LGR Height Extension (Autodesk Fusion 360 design; units mm, degrees)
Autodesk Fusion 360 part; units mm, degrees
note: some values were not read from the file. Set by a fixed rule: which sketch regions a step uses.
sketch "Sketch1" plane through (0, 0, 0) normal (0, 0, 1) x (1, 0, 0)
  line L0 (-28.575, 22.5) -> (28.575, 22.5)
  line L1 (28.575, 22.5) -> (28.575, -22.5)
  line L2 (28.575, -22.5) -> (-28.575, -22.5)
  line L3 (-28.575, -22.5) -> (-28.575, 22.5)
  dimension "d1" = 45
  dimension "d2" = 57.15
  dimension "d7" = 28.575
  dimension "d8" = 22.5
  constraint horizontal L0
  constraint vertical L1
  constraint horizontal L2
  constraint vertical L3
  measures "d1" distance of L0 L2
  measures "d2" distance of L1 L3
  measures "d7" distance of origin L1
  measures "d8" distance of origin L0
extrude "Extrude1" add sketch "Sketch1" along normal blind 1 makes body 1
sketch "Sketch3" plane through (0, 0, 1) normal (0, 0, 1) x (-1, 0, 0)
  line L0 (28.575, 22.5) -> (-28.575, 22.5)
  line L1 (-28.575, 22.5) -> (-28.575, -22.5)
  line L2 (-28.575, -22.5) -> (28.575, -22.5)
  line L3 (28.575, -22.5) -> (28.575, 22.5)
  line L4 (28.575, -22.5) -> (-28.575, -22.5)
  line L5 (-28.575, -22.5) -> (-28.575, -23.5)
  line L6 (-28.575, -23.5) -> (28.575, -23.5)
  line L7 (28.575, -23.5) -> (28.575, -22.5)
  dimension "d9" = 1
  dimension "d10" = 57.15
  constraint horizontal L4
  constraint vertical L5
  constraint horizontal L6
  constraint vertical L7
  constraint coincident L2.end L3.start
  measures "d9" distance of L4 L6
  measures "d10" distance of L5 L7
extrude "Extrude2" add sketch "Sketch3" along normal blind 45 separate body contours L2 L4 L5 L6 L7 makes body 2
extrude "Extrude3" add 1 faces at (-9.525, 23.1667, 1) along direction (0, 0, -1) blind 1 on bodies 2 bodies 1 2
extrude "Extrude4" add 1 faces at (9.525, 23.5, 30.6667) along direction (0, 1, 0) blind 5 on bodies 1 bodies 1
extrude "Extrude5" add 1 faces at (-9.525, 11.5, 0) along direction (0, 0, -1) blind 5 on bodies 1 bodies 1
sketch "Sketch5" plane through (0, 28.5, 0) normal (0, 1, 0) x (-1, 0, 0)
  line L0 (28.575, -5) -> (28.575, 46)
  line L1 (28.575, 46) -> (-28.575, 46)
  line L2 (-28.575, 46) -> (-28.575, -5)
  line L3 (-28.575, -5) -> (28.575, -5)
  point P0 (-20, 30.5)
  point P1 (20, 30.5)
  point P2 (-20, 18.5)
  point P3 (20, 18.5)
  dimension "d28" = 40
  dimension "d29" = 12
  dimension "d31" = 8.575
  dimension "d38" = 23.5
  constraint horizontal P0 P1
  constraint vertical P1 P3
  constraint horizontal P2 P3
  constraint vertical P0 P2
  measures "d28" distance of P0 P1
  measures "d29" distance of P1 P3
  measures "d31" distance of L2 P0
  measures "d38" distance of L3 P2
hole "Hole2" at (20, 28.5, 30.5) at (-20, 28.5, 30.5) at (-20, 28.5, 18.5) at (20, 28.5, 18.5) direction (0, -1, 0) diameter 5.5 depth 6 tip angle 180 counterbore diameter 10 counterbore depth 5 bodies 1
extrude "Extrude6" cut 1 faces at (-28.575, 9.5, -3) along direction (-1, 0, 0) blind 0 and the other way blind 2 on bodies 1 bodies 1
extrude "Extrude7" cut 1 faces at (28.575, 9.5, -3) along direction (1, 0, 0) blind 0 and the other way blind 2 on bodies 1 bodies 1
extrude "Extrude8" cut 1 faces at (-8.8583, 24.5, 46) along direction (0, 0, 1) blind 0 and the other way blind 7.5 on bodies 1 bodies 1
sketch "Sketch6" plane through (0, 28.5, 0) normal (0, 1, 0) x (-1, 0, 0)
  line L0 (26.575, 38.5) -> (-26.575, 38.5)
  line L1 (-26.575, 38.5) -> (-26.575, -5)
  line L2 (-26.575, -5) -> (26.575, -5)
  line L3 (26.575, -5) -> (26.575, 38.5)
  circle A0 centre (20, 18.5) radius 5
  circle A1 centre (-20, 30.5) radius 5
  circle A2 centre (20, 30.5) radius 5
  circle A3 centre (-20, 18.5) radius 5
  circle A4 centre (0, 24.5) radius 12.5
  dimension "d51" = 25
  dimension "d52" = 20
  dimension "d53" = 6
  measures "d51" diameter of A4
  measures "d52" horizontal distance of A3.centre A4.centre
  measures "d53" vertical distance of A2.centre A4.centre
extrude "Extrude9" cut sketch "Sketch6" along normal blind 0 and the other way blind 6 contours A4 bodies 1
sketch "Sketch9" plane through (0, 0, 1) normal (0, 0, 1) x (-1, 0, 0)
  line L0 (-26.575, 22.5) -> (-26.575, -22.5)
  line L1 (-26.575, -22.5) -> (26.575, -22.5)
  line L2 (26.575, -22.5) -> (26.575, 22.5)
  line L3 (26.575, 22.5) -> (-26.575, 22.5)
  line L4 (16.3972, -20) -> (-16.3972, -20)
  line L5 (24.075, -13.7886) -> (24.075, 13.7886)
  line L6 (16.3972, 20) -> (-16.3972, 20)
  line L7 (-24.075, 13.7886) -> (-24.075, -13.7886)
  line L8 (-1.2665, -3.0362) -> (-17.6637, -16.4521)
  line L9 (1.2665, -3.0362) -> (17.6637, -16.4521)
  line L10 (20.8111, -15.3386) -> (3.9009, -1.55)
  line L11 (3.9009, 1.55) -> (20.8111, 15.3386)
  line L12 (17.6637, 16.4521) -> (1.2665, 3.0362)
  line L13 (-1.2665, 3.0362) -> (-17.6637, 16.4521)
  line L14 (-20.8111, 15.3386) -> (-3.9009, 1.55)
  line L15 (-3.9009, -1.55) -> (-20.8111, -15.3386)
  arc A0 (20.8111, -15.3386) -> (24.075, -13.7886) centre (22.075, -13.7886) ccw
  arc A1 (3.9009, 1.55) -> (3.9009, -1.55) centre (5.1648, 0) ccw
  arc A2 (24.075, 13.7886) -> (20.8111, 15.3386) centre (22.075, 13.7886) ccw
  arc A3 (17.6637, 16.4521) -> (16.3972, 20) centre (16.3972, 18) ccw
  arc A4 (-16.3972, 20) -> (-17.6637, 16.4521) centre (-16.3972, 18) ccw
  arc A5 (-1.2665, 3.0362) -> (1.2665, 3.0362) centre (0, 4.5841) ccw
  arc A6 (-3.9009, -1.55) -> (-3.9009, 1.55) centre (-5.1648, 0) ccw
  arc A7 (-20.8111, 15.3386) -> (-24.075, 13.7886) centre (-22.075, 13.7886) ccw
  arc A8 (-24.075, -13.7886) -> (-20.8111, -15.3386) centre (-22.075, -13.7886) ccw
  arc A9 (-17.6637, -16.4521) -> (-16.3972, -20) centre (-16.3972, -18) ccw
  arc A10 (16.3972, -20) -> (17.6637, -16.4521) centre (16.3972, -18) ccw
  arc A11 (1.2665, -3.0362) -> (-1.2665, -3.0362) centre (0, -4.5841) ccw
  point P0 (22, -20)
  point P1 (-22, -20)
  point P2 (24.075, -18)
  point P3 (24.075, 18)
  point P4 (22, 20)
  point P5 (-22, 20)
  point P6 (-24.075, 18)
  point P7 (-24.075, -18)
  point P8 (0, -2)
  point P9 (-2, 0)
  point P10 (0, 2)
  point P11 (2, 0)
  dimension "d93" = 44
  dimension "d94" = 44
  dimension "d95" = 36
  dimension "d96" = 36
  dimension "d97" = 22
  dimension "d98" = 22
  dimension "d99" = 18
  dimension "d100" = 18
  dimension "d101" = 2.5
  dimension "d102" = 2.5
  dimension "d103" = 2.5
  dimension "d104" = 2.5
  dimension "d105" = 2
  dimension "d112" = 2
  constraint horizontal L4
  constraint parallel L2 L5
  constraint horizontal L6
  constraint parallel L0 L7
  constraint coincident P2 L10
  constraint coincident P2 L5
  constraint tangent L10 A0
  constraint tangent L5 A0
  constraint tangent L10 A1
  constraint tangent L11 A1
  constraint equal A0 A1
  constraint coincident P3 L11
  constraint coincident P3 L5
  constraint tangent L11 A2
  constraint tangent L5 A2
  constraint equal A0 A2
  constraint coincident P4 L12
  constraint coincident P4 L6
  constraint tangent L12 A3
  constraint tangent L6 A3
  constraint equal A0 A3
  constraint coincident P5 L6
  constraint coincident P5 L13
  constraint tangent L6 A4
  constraint tangent L13 A4
  constraint equal A0 A4
  constraint tangent L13 A5
  constraint tangent L12 A5
  constraint equal A0 A5
  constraint tangent L14 A6
  constraint tangent L15 A6
  constraint equal A0 A6
  constraint coincident P6 L14
  constraint coincident P6 L7
  constraint tangent L14 A7
  constraint tangent L7 A7
  constraint equal A0 A7
  constraint coincident P7 L7
  constraint coincident P7 L15
  constraint tangent L7 A8
  constraint tangent L15 A8
  constraint equal A0 A8
  constraint coincident P1 L8
  constraint coincident P1 L4
  constraint tangent L8 A9
  constraint tangent L4 A9
  constraint equal A0 A9
  constraint coincident P0 L9
  constraint coincident P0 L4
  constraint tangent L9 A10
  constraint tangent L4 A10
  constraint equal A0 A10
  constraint tangent L9 A11
  constraint tangent L8 A11
  measures "d93" distance of P0 P1
  measures "d94" distance of P4 P5
  measures "d95" distance of P6 P7
  measures "d96" distance of P2 P3
  measures "d97" horizontal distance of origin P1
  measures "d98" horizontal distance of origin P4
  measures "d99" vertical distance of origin P6
  measures "d100" vertical distance of origin P2
  measures "d101" distance of L3 L6
  measures "d102" distance of L0 L7
  measures "d103" distance of L2 L5
  measures "d104" distance of L1 L4
  measures "d105" radius of A0
  measures "d112" radius of A11
extrude "Extrude11" cut sketch "Sketch9" along normal blind 0 and the other way blind 6 contours L4 L8 L9 A9 A10 A11 | L5 L10 L11 A0 A1 A2 | L6 L12 L13 A3 A4 A5 | L7 L14 L15 A6 A7 A8 bodies 1
sketch "Sketch10" plane through (0, 22.5, 0) normal (0, -1, 0) x (1, 0, 0)
  circle A0 centre (0, 24.5) radius 12.5
  line L0 (26.575, 38.5) -> (-26.575, 38.5)
  line L1 (-26.575, 38.5) -> (-26.575, 1)
  line L2 (-26.575, 1) -> (26.575, 1)
  line L3 (26.575, 1) -> (26.575, 38.5)
  circle A1 centre (20, 18.5) radius 2.75
  circle A2 centre (-20, 30.5) radius 2.75
  circle A3 centre (20, 30.5) radius 2.75
  circle A4 centre (-20, 18.5) radius 2.75
  line L4 (-21.575, 9.5) -> (21.575, 9.5)
  line L5 (24.075, 7) -> (24.075, 6)
  line L6 (21.575, 3.5) -> (-21.575, 3.5)
  line L7 (-24.075, 6) -> (-24.075, 7)
  arc A5 (-21.575, 9.5) -> (-24.075, 7) centre (-21.575, 7) ccw
  arc A6 (-24.075, 6) -> (-21.575, 3.5) centre (-21.575, 6) ccw
  arc A7 (21.575, 3.5) -> (24.075, 6) centre (21.575, 6) ccw
  arc A8 (24.075, 7) -> (21.575, 9.5) centre (21.575, 7) ccw
  dimension "d113" = 2.5
  dimension "d114" = 2.5
  dimension "d115" = 2.5
  dimension "d116" = 15
  dimension "d117" = 2.5
  constraint horizontal L4
  constraint vertical L5
  constraint horizontal L6
  constraint vertical L7
  constraint tangent L4 A5
  constraint tangent L7 A5
  constraint tangent L7 A6
  constraint tangent L6 A6
  constraint equal A5 A6
  constraint tangent L6 A7
  constraint tangent L5 A7
  constraint equal A5 A7
  constraint tangent L5 A8
  constraint tangent L4 A8
  constraint equal A5 A8
  measures "d113" distance of L2 L6
  measures "d114" distance of L1 L7
  measures "d115" distance of L3 L5
  measures "d116" distance of A0.centre L4
  measures "d117" radius of A5
extrude "Extrude13" cut sketch "Sketch10" against normal blind 6 contours L4 L5 L6 L7 A5 A6 A7 A8 bodies 1
extrude "Extrude14" add 1 faces at (5.4657, 25.6667, -5) along direction (0, 0, -1) blind 5 on bodies 1 bodies 1
sketch "Sketch13" plane through (26.575, 0, 0) normal (1, 0, 0) x (0, 1, 0)
  line L0 (28.5, 38.5) -> (22.5, 38.5)
  line L1 (22.5, 38.5) -> (22.5, 1)
  line L2 (22.5, 1) -> (-22.5, 1)
  line L3 (-22.5, 1) -> (-22.5, -10)
  line L4 (-22.5, -10) -> (28.5, -10)
  line L5 (28.5, -10) -> (28.5, 38.5)
  line L6 (-13, -1.5) -> (13, -1.5)
  line L7 (15, -3.5) -> (15, -5.5)
  line L8 (13, -7.5) -> (-13, -7.5)
  line L9 (-15, -5.5) -> (-15, -3.5)
  arc A0 (-13, -1.5) -> (-15, -3.5) centre (-13, -3.5) ccw
  arc A1 (-15, -5.5) -> (-13, -7.5) centre (-13, -5.5) ccw
  arc A2 (13, -7.5) -> (15, -5.5) centre (13, -5.5) ccw
  arc A3 (15, -3.5) -> (13, -1.5) centre (13, -3.5) ccw
  dimension "d124" = 2.5
  dimension "d125" = 2.5
  dimension "d126" = 7.5
  dimension "d127" = 13.5
  dimension "d128" = 2
  constraint horizontal L6
  constraint vertical L7
  constraint horizontal L8
  constraint vertical L9
  constraint tangent L6 A0
  constraint tangent L9 A0
  constraint tangent L9 A1
  constraint tangent L8 A1
  constraint equal A0 A1
  constraint tangent L8 A2
  constraint tangent L7 A2
  constraint equal A0 A2
  constraint tangent L7 A3
  constraint tangent L6 A3
  constraint equal A0 A3
  measures "d124" distance of L2 L6
  measures "d125" distance of L4 L8
  measures "d126" distance of L3 L9
  measures "d127" distance of L5 L7
  measures "d128" radius of A0
extrude "Extrude15" cut sketch "Sketch13" against normal blind 4 contours L6 L7 L8 L9 A0 A1 A2 A3 bodies 1
sketch "Sketch14" plane through (0, -22.5, 0) normal (0, -1, 0) x (1, 0, 0)
  line L0 (26.575, -10) -> (26.575, 1)
  line L1 (26.575, 1) -> (-26.575, 1)
  line L2 (-26.575, 1) -> (-26.575, -10)
  line L3 (-26.575, -10) -> (26.575, -10)
  line L4 (-15.5, -1.5) -> (15.5, -1.5)
  line L5 (17.5, -3.5) -> (17.5, -5.5)
  line L6 (15.5, -7.5) -> (-15.5, -7.5)
  line L7 (-17.5, -5.5) -> (-17.5, -3.5)
  arc A0 (-15.5, -1.5) -> (-17.5, -3.5) centre (-15.5, -3.5) ccw
  arc A1 (-17.5, -5.5) -> (-15.5, -7.5) centre (-15.5, -5.5) ccw
  arc A2 (15.5, -7.5) -> (17.5, -5.5) centre (15.5, -5.5) ccw
  arc A3 (17.5, -3.5) -> (15.5, -1.5) centre (15.5, -3.5) ccw
  dimension "d131" = 2.5
  dimension "d132" = 2.5
  dimension "d133" = 9.075
  dimension "d134" = 9.075
  dimension "d135" = 2
  constraint horizontal L4
  constraint vertical L5
  constraint horizontal L6
  constraint vertical L7
  constraint tangent L4 A0
  constraint tangent L7 A0
  constraint tangent L7 A1
  constraint tangent L6 A1
  constraint equal A0 A1
  constraint tangent L6 A2
  constraint tangent L5 A2
  constraint equal A0 A2
  constraint tangent L4 A3
  constraint tangent L5 A3
  constraint equal A0 A3
  measures "d131" distance of L1 L4
  measures "d132" distance of L3 L6
  measures "d133" distance of L2 L7
  measures "d134" distance of L0 L5
  measures "d135" radius of A0
extrude "Extrude16" cut sketch "Sketch14" against normal blind 4 contours L4 L5 L6 L7 A0 A1 A2 A3 bodies 1
sketch "Sketch15" plane through (-26.575, 0, 0) normal (-1, 0, 0) x (0, -1, 0)
  line L0 (-22.5, 38.5) -> (-28.5, 38.5)
  line L1 (-28.5, 38.5) -> (-28.5, -10)
  line L2 (-28.5, -10) -> (22.5, -10)
  line L3 (22.5, -10) -> (22.5, 1)
  line L4 (22.5, 1) -> (-22.5, 1)
  line L5 (-22.5, 1) -> (-22.5, 38.5)
  line L6 (-13, -1.5) -> (13, -1.5)
  line L7 (15, -3.5) -> (15, -5.5)
  line L8 (13, -7.5) -> (-13, -7.5)
  line L9 (-15, -5.5) -> (-15, -3.5)
  arc A0 (15, -3.5) -> (13, -1.5) centre (13, -3.5) ccw
  arc A1 (13, -7.5) -> (15, -5.5) centre (13, -5.5) ccw
  arc A2 (-15, -5.5) -> (-13, -7.5) centre (-13, -5.5) ccw
  arc A3 (-13, -1.5) -> (-15, -3.5) centre (-13, -3.5) ccw
  dimension "d138" = 2.5
  dimension "d139" = 2.5
  dimension "d140" = 7.5
  dimension "d141" = 13.5
  dimension "d142" = 2
  constraint horizontal L6
  constraint vertical L7
  constraint horizontal L8
  constraint vertical L9
  constraint tangent L7 A0
  constraint tangent L6 A0
  constraint tangent L7 A1
  constraint tangent L8 A1
  constraint equal A0 A1
  constraint tangent L8 A2
  constraint tangent L9 A2
  constraint equal A0 A2
  constraint tangent L9 A3
  constraint tangent L6 A3
  constraint equal A0 A3
  measures "d138" distance of L4 L6
  measures "d139" distance of L2 L8
  measures "d140" distance of L3 L7
  measures "d141" distance of L1 L9
  measures "d142" radius of A0
extrude "Extrude17" cut sketch "Sketch15" against normal blind 4 contours L6 L7 L8 L9 A0 A1 A2 A3 bodies 1
sketch "Sketch16" plane through (0, 28.5, 0) normal (0, 1, 0) x (-1, 0, 0)
  line L0 (-24.075, 6) -> (-24.075, 7)
  arc A0 (-21.575, 9.5) -> (-24.075, 7) centre (-21.575, 7) ccw
  line L1 (-21.575, 9.5) -> (21.575, 9.5)
  arc A1 (24.075, 7) -> (21.575, 9.5) centre (21.575, 7) ccw
  line L2 (24.075, 7) -> (24.075, 6)
  arc A2 (21.575, 3.5) -> (24.075, 6) centre (21.575, 6) ccw
  line L3 (21.575, 3.5) -> (-21.575, 3.5)
  arc A3 (-24.075, 6) -> (-21.575, 3.5) centre (-21.575, 6) ccw
  circle A4 centre (0, 24.5) radius 12.5
  line L4 (26.575, 38.5) -> (-26.575, 38.5)
  line L5 (-26.575, 38.5) -> (-26.575, -10)
  line L6 (-26.575, -10) -> (26.575, -10)
  line L7 (26.575, -10) -> (26.575, 38.5)
  circle A5 centre (20, 18.5) radius 5
  circle A6 centre (-20, 30.5) radius 5
  circle A7 centre (20, 30.5) radius 5
  circle A8 centre (-20, 18.5) radius 5
  line L8 (-15.5, -1.5) -> (15.5, -1.5)
  line L9 (17.5, -3.5) -> (17.5, -5.5)
  line L10 (15.5, -7.5) -> (-15.5, -7.5)
  line L11 (-17.5, -5.5) -> (-17.5, -3.5)
  arc A9 (-15.5, -1.5) -> (-17.5, -3.5) centre (-15.5, -3.5) ccw
  arc A10 (-17.5, -5.5) -> (-15.5, -7.5) centre (-15.5, -5.5) ccw
  arc A11 (15.5, -7.5) -> (17.5, -5.5) centre (15.5, -5.5) ccw
  arc A12 (17.5, -3.5) -> (15.5, -1.5) centre (15.5, -3.5) ccw
  dimension "d145" = 5
  dimension "d146" = 2.5
  dimension "d147" = 9.075
  dimension "d148" = 9.075
  dimension "d149" = 2
  constraint horizontal L8
  constraint vertical L9
  constraint horizontal L10
  constraint vertical L11
  constraint tangent L8 A9
  constraint tangent L11 A9
  constraint tangent L11 A10
  constraint tangent L10 A10
  constraint equal A9 A10
  constraint tangent L10 A11
  constraint tangent L9 A11
  constraint equal A9 A11
  constraint tangent L9 A12
  constraint tangent L8 A12
  constraint equal A9 A12
  measures "d145" distance of L3 L8
  measures "d146" distance of L6 L10
  measures "d147" distance of L5 L11
  measures "d148" distance of L7 L9
  measures "d149" radius of A9
extrude "Extrude18" cut sketch "Sketch16" against normal blind 10 contours L8 L9 L10 L11 A9 A10 A11 A12 bodies 1
equation "d7 = ( 2.25 in / 2 )"
equation "d8 = ( 45 / 2 ) * 1 mm"
equation "d31 = ( 2.25 in - 40 mm ) / 2"
equation "d127 = 7.5 mm + 6 mm"
equation "d133 = ( ( 53.15 - 35 ) / 2 ) * 1 mm"
equation "d134 = ( ( 53.15 - 35 ) / 2 ) * 1 mm"
